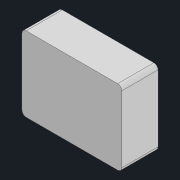
# Autodesk Inventor part: link0
Saved by Autodesk Inventor 2021 (Build 250183000, 183)
## iProperties
Created: 2021-07-10
Part Number: link0
Material: 一般
Document SubType Name: Modeling
Designer: yuta0
Density: 1 g/cm^3
Appearance: 既定
Author: yuta0
Autodesk Inventor part; units mm, degrees
ref_plane "YZ Plane" through (0, 0, 0) normal (1, 0, 0) x (0, 1, 0)
ref_plane "XZ Plane" through (0, 0, 0) normal (0, 1, 0) x (-1, 0, 0)
ref_plane "XY Plane" through (0, 0, 0) normal (0, 0, 1) x (1, 0, 0)
sketch "スケッチ1" plane through (0, 0, 0) normal (0, 0, 1) x (1, 0, 0)
  circle A0 centre (0, 0) radius 60
  line L0 (70, -90) -> (-170, -90)
  line L1 (-170, -90) -> (-170, 90)
  line L2 (-170, 90) -> (70, 90)
  line L3 (70, 90) -> (70, -90)
  line L4 (70, -90) -> (-170, 90) construction
  line L5 (-170, -90) -> (70, 90) construction
  point P0 (-50, 0)
  point P1 (-50, 0)
  point P2 (-50, 0)
  dimension "d0" = 120
  dimension "d3" = 240
  dimension "d4" = 180
  dimension "d10" = 70
  constraints: 12 end point, 4 midpoint, 2 parallel, 1 centre point, 1 coincident, 1 horizontal, 1 horizontal alignment, 1 perpendicular
  measures "d0" diameter of A0
  measures "d3" distance of L1.end L2.end
  measures "d4" distance of L0.end L1.end
  measures "d10" distance from line of L3 A0.centre
extrude "押し出し1" add sketch "スケッチ1" along normal blind 87 contours A0 | L0 L1 L2 L3
fillet "フィレット1" radius 10 4 edges at (70, 90, 43.5) (-170, 90, 43.5) (-170, -90, 43.5) (70, -90, 43.5)
